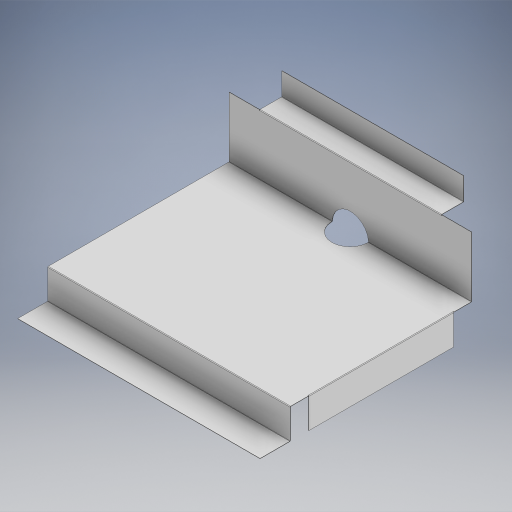
# Autodesk Inventor part: CE-3.1.2
Saved by Autodesk Inventor 2024 (Build 280153000, 153)
## iProperties
Created: 2024-02-01
Part Number: CE-3.1.2
Material: Generic
Document SubType Name: Sheet Metal
Designer: Alex
Density: 1 g/cm^3
Flat Pattern Width: 44.9131 cm
Flat Pattern Length: 57.0655 cm
Flat Pattern Area: 2562.99 cm^2
Sheet Metal Rule: Default_mm
Sheet Metal Width: 449.131 mm
Sheet Metal Length: 570.655 mm
Sheet Metal Area: 256298.776 mm^2
Appearance: Default
Author: Alex
Autodesk Inventor part; units mm, degrees
ref_plane "YZ Plane" through (0, 0, 0) normal (1, 0, 0) x (0, 1, 0)
ref_plane "XZ Plane" through (0, 0, 0) normal (0, 1, 0) x (-1, 0, 0)
ref_plane "XY Plane" through (0, 0, 0) normal (0, 0, 1) x (1, 0, 0)
sketch "Sketch1" plane through (0, 0, 0) normal (0, 1, 0) x (-1, 0, 0)
  line L0 (0, 0) -> (400, 0)
  line L1 (400, 0) -> (400, 300)
  line L2 (400, 300) -> (0, 300)
  line L3 (0, 300) -> (0, 0)
  dimension "d0" = 400
  dimension "d1" = 300
  measures "d0" distance of L2.end L1.end
  measures "d1" distance of L1.end L0.end
extrude "Plate1" add sketch "Sketch1" against normal blind 0.5
sketch "Sketch2" plane through (0, 0, 299.5) normal (0, 0, 1) x (1, 0, 0)
  line L0 (-400, 0) -> (0, 0)
  line L1 (0, 0) -> (0, 50)
  line L2 (0, 50) -> (-400, 50)
  line L3 (-400, 50) -> (-400, 0)
  constraints: 6 end point, 1 horizontal, 1 perpendicular, 1 vertical
edge flange "Flange1" height 50 angle 90 thickness 0.5 bend radius 0.5 thickness toward (0, 0, 1) relief straight relief width 0.5 relief depth 0.25 edges at (-200, 0, 300) wall of the first edge with corners at (-400, 0, 299.5) (0, 0, 299.5) (0, -50, 299.5) (-400, -50, 299.5)
bend "Bend1"
corner "Corner1"
sketch "Sketch3" plane through (0, -49.5, 299.5) normal (0, -1, 0) x (1, 0, 0)
  line L0 (-400, 0) -> (0, 0)
  line L1 (0, 0) -> (0, 50)
  line L2 (0, 50) -> (-400, 50)
  line L3 (-400, 50) -> (-400, 0)
  constraints: 6 end point, 1 horizontal, 1 perpendicular, 1 vertical
edge flange "Flange2" height 50 angle 90 thickness 0.5 bend radius 0.5 thickness toward (0, -1, 0) relief straight relief width 0.5 relief depth 0.25 edges at (-200, -50, 300) wall of the first edge with corners at (-400, -49.5, 299.5) (0, -49.5, 299.5) (0, -49.5, 349.5) (-400, -49.5, 349.5)
bend "Bend2"
corner "Corner2"
sketch "Sketch4" plane through (-0.5, 0, 0) normal (1, 0, 0) x (0, -1, 0)
  line L0 (0, 269) -> (0, 30)
  line L1 (0, 30) -> (50, 30)
  line L2 (50, 30) -> (50, 269)
  line L3 (50, 269) -> (0, 269)
  constraints: 8 end point
edge flange "Flange3" height 50 angle 90 thickness 0.5 bend radius 0.5 thickness toward (1, 0, 0) relief straight relief width 0.5 relief depth 0.25 edges at (0, 0, 149.5) wall of the first edge with corners at (-0.5, 0, 269) (-0.5, 0, 30) (-0.5, -50, 30) (-0.5, -50, 269)
bend "Bend3"
corner "Corner3"
sketch "Sketch5" plane through (-400, -0.5, 0.5) normal (0, 0, -1) x (-1, 0, 0)
  line L0 (-400, 0) -> (0, 0)
  line L1 (0, 0) -> (0, 100)
  line L2 (0, 100) -> (-400, 100)
  line L3 (-400, 100) -> (-400, 0)
  constraints: 6 end point, 1 horizontal, 1 perpendicular, 1 vertical
edge flange "Flange4" height 100 angle 90 thickness 0.5 bend radius 0.5 thickness toward (0, 0, -1) relief straight relief width 0.5 relief depth 0.25 edges at (-200, 0, 0) wall of the first edge with corners at (0, -0.5, 0.5) (-400, -0.5, 0.5) (-400, 99.5, 0.5) (0, 99.5, 0.5)
bend "Bend4"
corner "Corner4"
sketch "Sketch6" plane through (-400, 99, 0.5) normal (0, 1, 0) x (-1, 0, 0)
  line L0 (-350, 0) -> (-50, 0)
  line L1 (-50, 0) -> (-50, 37.5)
  line L2 (-50, 37.5) -> (-350, 37.5)
  line L3 (-350, 37.5) -> (-350, 0)
  constraints: 8 end point
edge flange "Flange5" height 37.5 angle 90 thickness 0.5 bend radius 0.5 thickness toward (0, 1, 0) relief straight relief width 0.5 relief depth 0.25 edges at (-200, 99.5, 0.5) wall of the first edge with corners at (-50, 99, 0.5) (-350, 99, 0.5) (-350, 99, -37) (-50, 99, -37)
bend "Bend5"
corner "Corner5"
sketch "Sketch7" plane through (-350, 99, -36.5) normal (0, 0, -1) x (-1, 0, 0)
  line L0 (-300, 0) -> (0, 0)
  line L1 (0, 0) -> (0, 37.5)
  line L2 (0, 37.5) -> (-300, 37.5)
  line L3 (-300, 37.5) -> (-300, 0)
  constraints: 6 end point, 1 horizontal, 1 perpendicular, 1 vertical
edge flange "Flange6" height 37.5 angle 90 thickness 0.5 bend radius 0.5 thickness toward (0, 0, -1) relief straight relief width 0.5 relief depth 0.25 edges at (-200, 99.5, -37) wall of the first edge with corners at (-50, 99, -36.5) (-350, 99, -36.5) (-350, 136.5, -36.5) (-50, 136.5, -36.5)
bend "Bend6"
corner "Corner6"
unfold all bends "Unfold1" k factor 0.44 fixed face at (-267.0833, 0, 189.6667)
sketch "Sketch8" plane through (0, 0, 0) normal (0, 1, 0) x (1, 0, 0)
  line L0 (0, -1) -> (-400, -1) projected
  circle A0 centre (-200, -1) radius 30
  point P0 (0, 0)
  dimension "d67" = 60
  constraints: 1 centre point, 1 midpoint
  measures "d67" diameter of A0
extrude "Cut1" cut sketch "Sketch8" against normal through all
refold all bends "Refold1"
equation "\"d68\" = Thickness"
equation "\"d2\" = Thickness"
equation "\"d3\" = BendReliefWidth"
equation "\"d4\" = BendReliefDepth"
equation "\"d5\" = MinimumRemnant"
equation "\"d6\" = TransitionRadius"
equation "\"d9\" = BendRadius"
equation "\"d10\" = CornerReliefSize"
equation "\"d11\" = GapSize"
equation "\"d12\" = JacobiRadiusSize"
equation "\"d13\" = BendReliefWidth"
equation "\"d14\" = BendReliefDepth"
equation "\"d15\" = MinimumRemnant"
equation "\"d16\" = TransitionRadius"
equation "\"d19\" = BendRadius"
equation "\"d20\" = CornerReliefSize"
equation "\"d21\" = GapSize"
equation "\"d22\" = JacobiRadiusSize"
equation "\"d23\" = BendReliefWidth"
equation "\"d24\" = BendReliefDepth"
equation "\"d25\" = MinimumRemnant"
equation "\"d26\" = TransitionRadius"
equation "\"d31\" = BendRadius"
equation "\"d32\" = CornerReliefSize"
equation "\"d33\" = GapSize"
equation "\"d34\" = JacobiRadiusSize"
equation "\"d35\" = BendReliefWidth"
equation "\"d36\" = BendReliefDepth"
equation "\"d37\" = MinimumRemnant"
equation "\"d38\" = TransitionRadius"
equation "\"d41\" = BendRadius"
equation "\"d42\" = CornerReliefSize"
equation "\"d43\" = GapSize"
equation "\"d44\" = JacobiRadiusSize"
equation "\"d45\" = BendReliefWidth"
equation "\"d46\" = BendReliefDepth"
equation "\"d47\" = MinimumRemnant"
equation "\"d48\" = TransitionRadius"
equation "\"d53\" = BendRadius"
equation "\"d54\" = CornerReliefSize"
equation "\"d55\" = GapSize"
equation "\"d56\" = JacobiRadiusSize"
equation "\"d57\" = BendReliefWidth"
equation "\"d58\" = BendReliefDepth"
equation "\"d59\" = MinimumRemnant"
equation "\"d60\" = TransitionRadius"
equation "\"d63\" = BendRadius"
equation "\"d64\" = CornerReliefSize"
equation "\"d65\" = GapSize"
equation "\"d66\" = JacobiRadiusSize"
equation "\"BendRadius\" = Thickness"
equation "\"BendReliefWidth\" = Thickness"
equation "\"BendReliefDepth\" = 0.5 * Thickness"
equation "\"CornerReliefSize\" = 4 * Thickness"
equation "\"MinimumRemnant\" = 2 * Thickness"
equation "\"TransitionRadius\" = BendRadius"
equation "\"JacobiRadiusSize\" = BendRadius"
equation "\"GapSize\" = Thickness"
equation "\"Thickness\" = 0.5"
body "Solid1"
